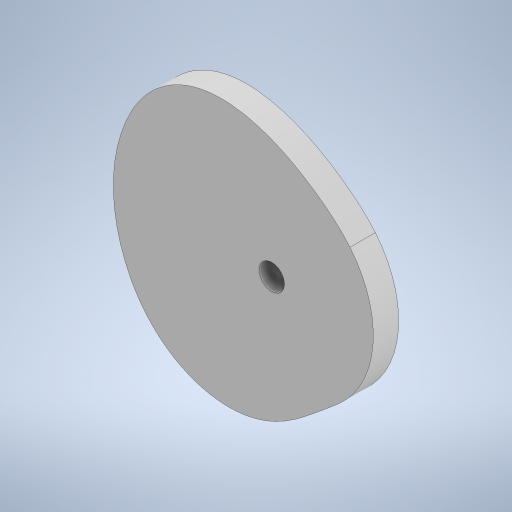
# Autodesk Inventor part: 凸輪_4
Saved by Autodesk Inventor 2023 (Build 270158000, 158)
## iProperties
Created: 2023-05-17
Part Number: 凸輪_4
Material: 一般
Document SubType Name: Modeling
Designer: JOU
Density: 1 g/cm^3
Appearance: 預設
Author: JOU
Autodesk Inventor part; units mm, degrees
ref_plane "YZ Plane" through (0, 0, 0) normal (1, 0, 0) x (0, 1, 0)
ref_plane "XZ Plane" through (0, 0, 0) normal (0, 1, 0) x (-1, 0, 0)
ref_plane "XY Plane" through (0, 0, 0) normal (0, 0, 1) x (1, 0, 0)
sketch "草圖1" plane through (0, 0, 0) normal (0, 0, 1) x (1, 0, 0)
  spline S0 degree 5 poles (30.808, 25.5122) (30.7, 25.6427) (30.5185, 25.8598) (30.2427, 26.1842) (29.8683, 26.6138) (29.3893, 27.1463) (28.9189, 27.6542) (28.418, 28.1797) (27.9061, 28.7018) (27.3833, 29.2208) (26.85, 29.7368) (26.3062, 30.2498) (25.7523, 30.76) (25.1883, 31.2674) (24.6146, 31.7722) (24.0311, 32.2744) (23.4381, 32.7742) (22.8357, 33.2715) (22.2241, 33.7665) (21.6033, 34.2591) (20.9735, 34.7494) (20.3347, 35.2374) (19.6871, 35.7231) (19.0306, 36.2064) (18.3654, 36.6872) (17.6914, 37.1655) (17.0087, 37.6412) (16.3174, 38.1142) (15.6173, 38.5843) (14.9086, 39.0513) (14.1912, 39.5151) (13.4652, 39.9754) (12.7304, 40.432) (11.987, 40.8847) (11.2348, 41.3331) (10.4739, 41.777) (9.7043, 42.2161) (8.9259, 42.6499) (8.1389, 43.0781) (7.3432, 43.5004) (6.5388, 43.9162) (5.7259, 44.3252) (4.9044, 44.727) (4.0745, 45.1211) (3.2362, 45.5069) (2.3896, 45.884) (1.535, 46.252) (0.6724, 46.6102) (-0.198, 46.9581) (-1.076, 47.2953) (-1.9614, 47.6211) (-2.8539, 47.9351) (-3.7532, 48.2366) (-4.6592, 48.5251) (-5.5715, 48.8002) (-6.4898, 49.0611) (-7.4137, 49.3075) (-8.343, 49.5386) (-9.2771, 49.7541) (-10.2159, 49.9534) (-11.1587, 50.136) (-12.1053, 50.3013) (-13.0552, 50.449) (-14.008, 50.5785) (-14.9632, 50.6893) (-15.9203, 50.7811) (-16.879, 50.8534) (-17.8387, 50.9059) (-18.7989, 50.938) (-19.7593, 50.9496) (-20.7192, 50.9402) (-21.6782, 50.9095) (-22.6359, 50.8572) (-23.5918, 50.7831) (-24.5453, 50.6869) (-25.4961, 50.5683) (-26.4435, 50.4271) (-27.3873, 50.2632) (-28.3268, 50.0764) (-29.2616, 49.8665) (-30.1912, 49.6334) (-31.1153, 49.377) (-32.0333, 49.0971) (-32.9447, 48.7938) (-33.8491, 48.467) (-34.7461, 48.1166) (-35.6352, 47.7427) (-36.5159, 47.3452) (-37.3878, 46.9243) (-38.2504, 46.4799) (-39.1032, 46.0121) (-39.9459, 45.5212) (-40.7779, 45.0072) (-41.5989, 44.4702) (-42.4083, 43.9106) (-43.2058, 43.3284) (-43.9909, 42.724) (-44.7631, 42.0976) (-45.5222, 41.4494) (-46.2676, 40.78) (-46.9989, 40.0895) (-47.7159, 39.3784) (-48.4181, 38.647) (-49.1051, 37.8958) (-49.7768, 37.1253) (-50.4327, 36.3359) (-51.0726, 35.5281) (-51.6962, 34.7023) (-52.3034, 33.8592) (-52.8938, 32.9993) (-53.4673, 32.1231) (-54.0239, 31.2311) (-54.5632, 30.3239) (-55.0854, 29.4021) (-55.5903, 28.4663) (-56.0778, 27.517) (-56.5481, 26.5547) (-57.001, 25.5802) (-57.4368, 24.5938) (-57.8553, 23.5963) (-58.2567, 22.5885) (-58.6412, 21.5706) (-59.0085, 20.5446) (-59.3579, 19.5122) (-59.6894, 18.4734) (-60.0027, 17.4289) (-60.2977, 16.379) (-60.5744, 15.3242) (-60.8326, 14.2647) (-61.0723, 13.2009) (-61.2934, 12.133) (-61.4958, 11.0614) (-61.6795, 9.9865) (-61.8443, 8.9085) (-61.9904, 7.8278) (-62.1176, 6.7448) (-62.2258, 5.6596) (-62.3151, 4.5728) (-62.3854, 3.4845) (-62.4368, 2.3952) (-62.469, 1.3052) (-62.4823, 0.2148) (-62.4765, -0.8757) (-62.4517, -1.966) (-62.4079, -3.0556) (-62.3451, -4.1443) (-62.2633, -5.2318) (-62.1625, -6.3176) (-62.0427, -7.4015) (-61.9041, -8.4832) (-61.7466, -9.5623) (-61.5704, -10.6384) (-61.3753, -11.7114) (-61.1616, -12.7807) (-60.9292, -13.8462) (-60.6783, -14.9075) (-60.4089, -15.9642) (-60.121, -17.016) (-59.8149, -18.0627) (-59.4905, -19.104) (-59.1479, -20.1399) (-58.7871, -21.1698) (-58.4079, -22.1948) (-58.0091, -23.2159) (-57.5904, -24.2322) (-57.1511, -25.2436) (-56.6908, -26.2493) (-56.209, -27.2488) (-55.7052, -28.2414) (-55.1793, -29.2264) (-54.6307, -30.203) (-54.0594, -31.1705) (-53.4649, -32.1279) (-52.8473, -33.0746) (-52.2063, -34.0097) (-51.5419, -34.9321) (-50.854, -35.8412) (-50.1428, -36.7359) (-49.4082, -37.6154) (-48.6506, -38.4787) (-47.8699, -39.3249) (-47.0667, -40.1531) (-46.2411, -40.9623) (-45.3937, -41.7516) (-44.5248, -42.5201) (-43.635, -43.267) (-42.7248, -43.9912) (-41.795, -44.692) (-40.8462, -45.3685) (-39.8793, -46.02) (-38.8949, -46.6455) (-37.8941, -47.2444) (-36.8776, -47.816) (-35.8466, -48.3596) (-34.8021, -48.8746) (-33.7451, -49.3603) (-32.6767, -49.8164) (-31.5981, -50.2423) (-30.5104, -50.6376) (-29.415, -51.002) (-28.313, -51.3352) (-27.2057, -51.6371) (-26.0943, -51.9074) (-24.9802, -52.1462) (-23.8645, -52.3534) (-22.7488, -52.5291) (-21.634, -52.6735) (-20.5217, -52.7869) (-19.413, -52.8694) (-18.3091, -52.9216) (-17.2112, -52.9439) (-16.1205, -52.9367) (-15.0382, -52.9008) (-13.9653, -52.8368) (-12.9029, -52.7454) (-11.8519, -52.6274) (-10.8132, -52.4836) (-9.7879, -52.3151) (-8.7766, -52.1226) (-7.7801, -51.9073) (-6.7992, -51.6701) (-5.8343, -51.4122) (-4.8861, -51.1345) (-3.9551, -50.8384) (-3.0415, -50.5248) (-2.1458, -50.195) (-1.2681, -49.85) (-0.4087, -49.4912) (0.4323, -49.1196) (1.255, -48.7363) (2.0593, -48.3426) (2.8454, -47.9395) (3.6134, -47.5281) (4.3635, -47.1094) (5.0961, -46.6846) (5.8116, -46.2546) (6.5102, -45.8203) (7.1926, -45.3826) (7.8591, -44.9424) (8.5103, -44.5006) (9.1468, -44.0578) (9.7692, -43.6147) (10.3782, -43.172) (10.9744, -42.7304) (11.5586, -42.2902) (12.1314, -41.8519) (12.6936, -41.416) (13.2459, -40.9828) (13.7891, -40.5525) (14.3239, -40.1254) (14.8511, -39.7015) (15.3713, -39.281) (15.8854, -38.8638) (16.3941, -38.4499) (16.898, -38.0391) (17.3978, -37.6314) (17.8941, -37.2264) (18.3876, -36.8238) (18.8788, -36.4232) (19.3682, -36.0244) (19.8563, -35.6267) (20.3436, -35.2297) (20.8304, -34.8328) (21.317, -34.4354) (21.8037, -34.0369) (22.2906, -33.6366) (22.778, -33.2339) (23.2658, -32.8281) (23.7541, -32.4184) (24.2428, -32.0041) (24.7317, -31.5846) (25.2206, -31.1591) (25.7093, -30.7269) (26.1973, -30.2874) (26.6844, -29.8399) (27.17, -29.3839) (27.6537, -28.9187) (28.1348, -28.4438) (28.6127, -27.9588) (29.0868, -27.4632) (29.5558, -26.9572) (30.0196, -26.4399) (30.4758, -25.9127) (30.9228, -25.3776) (31.3609, -24.8342) (31.7895, -24.2831) (32.2085, -23.7246) (32.6176, -23.1589) (33.0168, -22.5861) (33.406, -22.0064) (33.785, -21.4201) (34.1537, -20.8272) (34.5119, -20.2279) (34.8597, -19.6225) (35.1969, -19.0112) (35.5233, -18.394) (35.8389, -17.7712) (36.1436, -17.143) (36.4373, -16.5096) (36.7199, -15.8712) (36.9913, -15.2279) (37.2514, -14.58) (37.5002, -13.9277) (37.7375, -13.2711) (37.9634, -12.6105) (38.1777, -11.946) (38.3804, -11.2779) (38.5714, -10.6063) (38.7506, -9.9316) (38.918, -9.2538) (39.0736, -8.5731) (39.2173, -7.8899) (39.349, -7.2043) (39.4687, -6.5164) (39.5764, -5.8266) (39.6721, -5.135) (39.7557, -4.4419) (39.8271, -3.7474) (39.8865, -3.0517) (39.9337, -2.3551) (39.9687, -1.6578) (39.9915, -0.96) (40.0022, -0.2619) (40.0007, 0.4362) (39.987, 1.1343) (39.9611, 1.832) (39.923, 2.5291) (39.8728, 3.2255) (39.8104, 3.9209) (39.7359, 4.6151) (39.6493, 5.3078) (39.5507, 5.999) (39.4399, 6.6884) (39.3172, 7.3757) (39.1825, 8.0607) (39.0359, 8.7433) (38.8773, 9.4233) (38.7069, 10.1003) (38.5248, 10.7743) (38.3309, 11.445) (38.1253, 12.1122) (37.9081, 12.7758) (37.6793, 13.4354) (37.4391, 14.091) (37.1875, 14.7422) (36.9246, 15.389) (36.6504, 16.0311) (36.365, 16.6683) (36.0686, 17.3004) (35.7611, 17.9272) (35.4428, 18.5486) (35.1137, 19.1644) (34.7739, 19.7743) (34.4235, 20.3781) (34.0626, 20.9758) (33.6913, 21.5671) (33.3098, 22.1518) (32.9181, 22.7297) (32.5164, 23.3008) (32.1212, 23.8422) (31.7001, 24.3996) (31.3557, 24.8392) (31.0927, 25.1659) (30.9153, 25.3826) (30.808, 25.5122) knots 0 0 0 0 0 0 0.002983 0.004977 0.007475 0.009981 0.012497 0.015022 0.017556 0.020099 0.022652 0.025214 0.027786 0.030367 0.032958 0.035558 0.038167 0.040786 0.043415 0.046052 0.0487 0.051356 0.054022 0.056697 0.059381 0.062074 0.064777 0.067488 0.070208 0.072937 0.075674 0.078421 0.081175 0.083938 0.086709 0.089488 0.092276 0.09507 0.097873 0.100682 0.103499 0.106322 0.109152 0.111988 0.114831 0.117679 0.120532 0.123391 0.126254 0.129122 0.131994 0.134869 0.137748 0.14063 0.143515 0.146402 0.149291 0.152182 0.155074 0.157968 0.160862 0.163757 0.166652 0.169547 0.172442 0.175337 0.178231 0.181125 0.184019 0.186912 0.189804 0.192695 0.195586 0.198476 0.201366 0.204256 0.207145 0.210035 0.212925 0.215815 0.218706 0.221599 0.224492 0.227388 0.230285 0.233184 0.236087 0.238992 0.2419 0.244812 0.247727 0.250647 0.253571 0.2565 0.259434 0.262373 0.265317 0.268266 0.271221 0.274182 0.277149 0.280122 0.283101 0.286086 0.289077 0.292074 0.295077 0.298087 0.301102 0.304123 0.307151 0.310184 0.313223 0.316267 0.319317 0.322373 0.325433 0.328499 0.33157 0.334646 0.337725 0.340806 0.343889 0.346972 0.350055 0.353138 0.356222 0.359305 0.362388 0.365471 0.368555 0.371638 0.374721 0.377804 0.380887 0.383971 0.387054 0.390137 0.39322 0.396304 0.399387 0.40247 0.405553 0.408637 0.41172 0.414803 0.417886 0.420969 0.424053 0.427136 0.430219 0.433302 0.436386 0.439469 0.442552 0.445635 0.448719 0.451802 0.454885 0.457969 0.461054 0.464141 0.467232 0.470328 0.473428 0.476533 0.479643 0.482758 0.485878 0.489002 0.492132 0.495266 0.498405 0.501549 0.504697 0.507849 0.511005 0.514166 0.51733 0.520498 0.523669 0.526843 0.53002 0.5332 0.536382 0.539566 0.542752 0.545939 0.549127 0.552315 0.555503 0.558691 0.561879 0.565065 0.568249 0.571431 0.57461 0.577786 0.580958 0.584126 0.587289 0.590446 0.593597 0.596742 0.59988 0.60301 0.606132 0.609244 0.612348 0.615442 0.618525 0.621597 0.624658 0.627706 0.630743 0.633766 0.636775 0.63977 0.642751 0.645717 0.648668 0.651602 0.65452 0.657422 0.660306 0.663173 0.666022 0.668853 0.671666 0.67446 0.677234 0.67999 0.682727 0.685444 0.688141 0.690819 0.693477 0.696116 0.698735 0.701335 0.703915 0.706477 0.70902 0.711545 0.714053 0.716543 0.719017 0.721475 0.723918 0.726346 0.728761 0.731164 0.733555 0.735936 0.738307 0.74067 0.743027 0.745378 0.747724 0.750067 0.752408 0.754748 0.757088 0.75943 0.761775 0.764122 0.766475 0.768832 0.771195 0.773565 0.775942 0.778327 0.78072 0.783121 0.785531 0.78795 0.790377 0.792814 0.795259 0.797712 0.800171 0.802635 0.805101 0.807568 0.810035 0.812502 0.814969 0.817436 0.819903 0.82237 0.824837 0.827304 0.829771 0.832238 0.834705 0.837173 0.83964 0.842107 0.844574 0.847041 0.849508 0.851975 0.854442 0.856909 0.859376 0.861843 0.86431 0.866777 0.869244 0.871711 0.874178 0.876645 0.879112 0.881579 0.884046 0.886513 0.88898 0.891447 0.893914 0.896381 0.898848 0.901315 0.903782 0.906249 0.908716 0.911183 0.91365 0.916117 0.918584 0.921051 0.923518 0.925985 0.928452 0.930919 0.933386 0.935853 0.93832 0.940787 0.943254 0.945721 0.948188 0.950655 0.953122 0.955589 0.958056 0.960523 0.96299 0.965458 0.967925 0.970392 0.972859 0.975326 0.977793 0.98026 0.982727 0.985194 0.987661 0.990128 0.992595 0.995063 0.997037 1 1 1 1 1 1
  circle A0 centre (0, 0) radius 5
  point P0 (29.8876, 26.5879)
  point P1 (29.4096, 27.1202)
  point P2 (28.9202, 27.6491)
  point P3 (28.4194, 28.1746)
  point P4 (27.9077, 28.6968)
  point P5 (27.3851, 29.2158)
  point P6 (26.8519, 29.7318)
  point P7 (26.3082, 30.2448)
  point P8 (25.7544, 30.7551)
  point P9 (25.1906, 31.2625)
  point P10 (24.6169, 31.7674)
  point P11 (24.0335, 32.2697)
  point P12 (23.4406, 32.7695)
  point P13 (22.8383, 33.2669)
  point P14 (22.2268, 33.7619)
  point P15 (21.6061, 34.2546)
  point P16 (20.9763, 34.745)
  point P17 (20.3376, 35.233)
  point P18 (19.69, 35.7187)
  point P19 (19.0335, 36.202)
  point P20 (18.3683, 36.6829)
  point P21 (17.6944, 37.1612)
  point P22 (17.0117, 37.637)
  point P23 (16.3204, 38.11)
  point P24 (15.6203, 38.5801)
  point P25 (14.9116, 39.0471)
  point P26 (14.1942, 39.5109)
  point P27 (13.4682, 39.9712)
  point P28 (12.7334, 40.4279)
  point P29 (11.9899, 40.8806)
  point P30 (11.2377, 41.329)
  point P31 (10.4767, 41.7729)
  point P32 (9.707, 42.212)
  point P33 (8.9286, 42.6458)
  point P34 (8.1415, 43.0741)
  point P35 (7.3457, 43.4963)
  point P36 (6.5413, 43.9122)
  point P37 (5.7282, 44.3212)
  point P38 (4.9066, 44.723)
  point P39 (4.0765, 45.1171)
  point P40 (3.2381, 45.5029)
  point P41 (2.3914, 45.88)
  point P42 (1.5366, 46.248)
  point P43 (0.6739, 46.6062)
  point P44 (-0.1967, 46.9541)
  point P45 (-1.0748, 47.2913)
  point P46 (-1.9603, 47.6171)
  point P47 (-2.853, 47.931)
  point P48 (-3.7525, 48.2326)
  point P49 (-4.6586, 48.5211)
  point P50 (-5.5711, 48.7961)
  point P51 (-6.4895, 49.057)
  point P52 (-7.4136, 49.3033)
  point P53 (-8.3429, 49.5344)
  point P54 (-9.2772, 49.7499)
  point P55 (-10.2161, 49.9491)
  point P56 (-11.159, 50.1316)
  point P57 (-12.1057, 50.2968)
  point P58 (-13.0557, 50.4444)
  point P59 (-14.0085, 50.5738)
  point P60 (-14.9638, 50.6846)
  point P61 (-15.9209, 50.7763)
  point P62 (-16.8796, 50.8485)
  point P63 (-17.8392, 50.9008)
  point P64 (-18.7994, 50.9329)
  point P65 (-19.7596, 50.9443)
  point P66 (-20.7195, 50.9348)
  point P67 (-21.6784, 50.9041)
  point P68 (-22.6359, 50.8517)
  point P69 (-23.5916, 50.7775)
  point P70 (-24.5449, 50.6812)
  point P71 (-25.4955, 50.5626)
  point P72 (-26.4427, 50.4214)
  point P73 (-27.3861, 50.2575)
  point P74 (-28.3254, 50.0707)
  point P75 (-29.2599, 49.8608)
  point P76 (-30.1893, 49.6277)
  point P77 (-31.113, 49.3713)
  point P78 (-32.0307, 49.0916)
  point P79 (-32.9418, 48.7884)
  point P80 (-33.8459, 48.4616)
  point P81 (-34.7426, 48.1114)
  point P82 (-35.6313, 47.7376)
  point P83 (-36.5117, 47.3403)
  point P84 (-37.3833, 46.9195)
  point P85 (-38.2456, 46.4753)
  point P86 (-39.0982, 46.0078)
  point P87 (-39.9406, 45.517)
  point P88 (-40.7724, 45.0032)
  point P89 (-41.5931, 44.4665)
  point P90 (-42.4023, 43.9071)
  point P91 (-43.1996, 43.3252)
  point P92 (-43.9845, 42.721)
  point P93 (-44.7566, 42.0948)
  point P94 (-45.5155, 41.4469)
  point P95 (-46.2608, 40.7777)
  point P96 (-46.9921, 40.0875)
  point P97 (-47.709, 39.3766)
  point P98 (-48.4111, 38.6454)
  point P99 (-49.0982, 37.8945)
  point P100 (-49.7698, 37.1242)
  point P101 (-50.4257, 36.335)
  point P102 (-51.0656, 35.5273)
  point P103 (-51.6893, 34.7018)
  point P104 (-52.2965, 33.8589)
  point P105 (-52.887, 32.9991)
  point P106 (-53.4606, 32.123)
  point P107 (-54.0172, 31.2312)
  point P108 (-54.5567, 30.3241)
  point P109 (-55.0789, 29.4025)
  point P110 (-55.5839, 28.4668)
  point P111 (-56.0716, 27.5176)
  point P112 (-56.5419, 26.5554)
  point P113 (-56.995, 25.5809)
  point P114 (-57.4309, 24.5947)
  point P115 (-57.8497, 23.5971)
  point P116 (-58.2514, 22.5888)
  point P117 (-58.6362, 21.5704)
  point P118 (-59.0038, 20.5437)
  point P119 (-59.3533, 19.5109)
  point P120 (-59.6848, 18.472)
  point P121 (-59.9981, 17.4276)
  point P122 (-60.2931, 16.3778)
  point P123 (-60.5698, 15.3231)
  point P124 (-60.828, 14.2636)
  point P125 (-61.0676, 13.1999)
  point P126 (-61.2887, 12.1321)
  point P127 (-61.4911, 11.0606)
  point P128 (-61.6748, 9.9857)
  point P129 (-61.8396, 8.9078)
  point P130 (-61.9857, 7.8272)
  point P131 (-62.1128, 6.7442)
  point P132 (-62.2211, 5.6592)
  point P133 (-62.3104, 4.5724)
  point P134 (-62.3807, 3.4843)
  point P135 (-62.432, 2.395)
  point P136 (-62.4643, 1.3051)
  point P137 (-62.4776, 0.2147)
  point P138 (-62.4718, -0.8757)
  point P139 (-62.447, -1.9658)
  point P140 (-62.4032, -3.0554)
  point P141 (-62.3403, -4.144)
  point P142 (-62.2585, -5.2314)
  point P143 (-62.1577, -6.3171)
  point P144 (-62.038, -7.401)
  point P145 (-61.8994, -8.4825)
  point P146 (-61.7419, -9.5615)
  point P147 (-61.5657, -10.6376)
  point P148 (-61.3706, -11.7105)
  point P149 (-61.1569, -12.7798)
  point P150 (-60.9246, -13.8452)
  point P151 (-60.6737, -14.9063)
  point P152 (-60.4043, -15.963)
  point P153 (-60.1165, -17.0147)
  point P154 (-59.8104, -18.0613)
  point P155 (-59.486, -19.1024)
  point P156 (-59.1436, -20.1377)
  point P157 (-58.7831, -21.1668)
  point P158 (-58.4041, -22.191)
  point P159 (-58.0055, -23.2114)
  point P160 (-57.5868, -24.2275)
  point P161 (-57.1475, -25.2386)
  point P162 (-56.6871, -26.2441)
  point P163 (-56.2052, -27.2435)
  point P164 (-55.7015, -28.236)
  point P165 (-55.1755, -29.2208)
  point P166 (-54.627, -30.1973)
  point P167 (-54.0556, -31.1647)
  point P168 (-53.4612, -32.1221)
  point P169 (-52.8435, -33.0686)
  point P170 (-52.2025, -34.0036)
  point P171 (-51.5381, -34.926)
  point P172 (-50.8503, -35.8349)
  point P173 (-50.139, -36.7296)
  point P174 (-49.4045, -37.609)
  point P175 (-48.6468, -38.4722)
  point P176 (-47.8662, -39.3184)
  point P177 (-47.0629, -40.1465)
  point P178 (-46.2374, -40.9557)
  point P179 (-45.3899, -41.745)
  point P180 (-44.521, -42.5135)
  point P181 (-43.6311, -43.2603)
  point P182 (-42.721, -43.9845)
  point P183 (-41.7911, -44.6853)
  point P184 (-40.8423, -45.3618)
  point P185 (-39.8753, -46.0133)
  point P186 (-38.8908, -46.6388)
  point P187 (-37.8899, -47.2377)
  point P188 (-36.8734, -47.8093)
  point P189 (-35.8423, -48.3529)
  point P190 (-34.7977, -48.8679)
  point P191 (-33.7405, -49.3537)
  point P192 (-32.672, -49.8097)
  point P193 (-31.5933, -50.2356)
  point P194 (-30.5055, -50.6309)
  point P195 (-29.41, -50.9953)
  point P196 (-28.3078, -51.3285)
  point P197 (-27.2003, -51.6303)
  point P198 (-26.0888, -51.9006)
  point P199 (-24.9745, -52.1394)
  dimension "d0" = 10
  constraints: 1 centre point, 1 coincident, 360 other
  measures "d0" diameter of A0
extrude "擠出1" add sketch "草圖1" along normal blind 10
